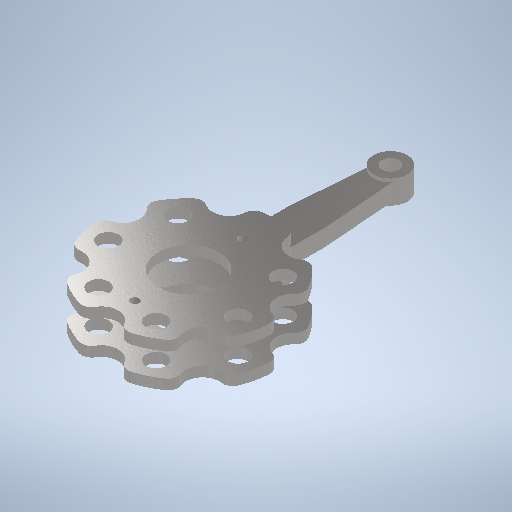
# Autodesk Inventor part: ring
Saved by Autodesk Inventor 2025 (Build 290162010, 162A)
## iProperties
Created: 2024-03-13
Part Number: ring
Material: Stahl, galvanisiert
Document SubType Name: Modeling
Designer: ffogue
Density: 7.85 g/cm^3
Appearance: Galvanisiert
Author: ffogue
Autodesk Inventor part; units mm, degrees
note: some values were not read from the file. Chosen so that the rebuilt part matches the saved one: direction of "Bohrung4"; direction of "Bohrung5"; direction of "Bohrung9"; direction of "Bohrung8".
sketch "Skizze13" plane through (0, 0, 0) normal (0, 1, 0) x (-1, 0, 0)
  line L0 (-5, 6.5) -> (5, 6.5)
  line L1 (5, 6.5) -> (5, -6.5)
  line L2 (5, -6.5) -> (-5, -6.5)
  line L3 (-5, -6.5) -> (-5, 6.5)
  line L4 (-5, 6.5) -> (5, -6.5) construction
  line L5 (5, 6.5) -> (-5, -6.5) construction
  point P0 (0, 0)
  point P1 (0, -6.5)
  dimension "d62" = 13
  dimension "d63" = 10
  constraints: 12 end point, 3 midpoint, 2 parallel, 1 horizontal, 1 perpendicular
  measures "d62" distance from line of point (0, -6.5) L0
  measures "d63" distance between parallel lines of L3 L1
extrude "Extrusion7" add sketch "Skizze13" along normal blind 5
ref_plane "Arbeitsebene3" through (0, 0, 0) normal (0, 0, 1) x (1, 0, 0)
sketch "Skizze14" plane through (0, 0, 0) normal (0, 0, 1) x (1, 0, 0)
  circle A0 centre (0, -20.5147) radius 26
  point P0 (0, 0)
  point P1 (-5, 5)
  point P2 (5, 5)
  dimension "d68" = 52
  constraints: 2 point on circle, 1 centre point
  measures "d68" diameter of A0
extrude "Extrusion8" add sketch "Skizze14" along normal mid plane 13
ref_plane "Arbeitsebene8" through (0, 0, 0) normal (0, 0, 1) x (1, 0, 0)
sketch "Skizze16" plane through (0, 5, 0) normal (0, 0, 1) x (1, 0, 0)
  line L0 (-5.4606, -0.0946) -> (-5.4606, 9.9054)
  line L1 (5.4606, -0.0946) -> (5.4606, 9.9054)
  line L2 (-5.4606, 9.9054) -> (-3.5, 34.4853)
  line L3 (-3.5, 34.4853) -> (3.5, 34.4853)
  line L4 (3.5, 34.4853) -> (5.4606, 9.9054)
  circle A0 centre (0, -25.5147) radius 26 projected
  line L5 (-5.4606, -0.0946) -> (5.4606, -0.0946)
  point P0 (0, 34.4853)
  point P1 (0, 0)
  point P2 (0, -0.0946)
  dimension "d75" = 7
  dimension "d76" = 60
  dimension "d77" = 175.44
  dimension "d153" = 10
  constraints: 13 end point, 2 horizontal, 2 midpoint, 2 vertical, 2 vertical alignment, 1 equal length, 1 horizontal alignment, 2 other
  measures "d75" distance of L2.end L3.end
  measures "d76" distance from line of point (0, -25.515) L3
  measures "d77" angle of L1 L4
  measures "d153" distance of L0.start L0.end
extrude "Extrusion10" add sketch "Skizze16" along normal mid plane 5 contours L0 L2 L3 L4 L1 A0 | A0 L5 picked at (-0.6108, 0.0772)
ref_plane "Arbeitsebene9" through (0, 0, 0) normal (0, 0, 1) x (1, 0, 0)
sketch "Skizze17" plane through (0, -20.5147, 0) normal (0, 0, 1) x (1, 0, 0)
  circle A0 centre (0, 60) radius 5
  line L0 (-3.5, 60) -> (3.5, 60) projected
  point P0 (0, 20.5147)
  dimension "d129" = 10
  constraints: 1 coincident, 1 horizontal alignment, 1 midpoint, 1 other
extrude "Extrusion11" add sketch "Skizze17" along normal mid plane 7
sketch "Skizze18" plane through (0, -20.5147, 6.5) normal (0, 0, 1) x (1, 0, 0)
  circle A0 centre (0, 60) radius 5 projected
  point P0 (0, 20.5147)
  point P1 (0, 60)
  point P2 (3.5, 60)
  point P3 (-3.5, 60)
  point P4 (3.7626, 56.7072)
  point P5 (-3.7626, 56.7072)
  constraints: 1 coincident
hole "Bohrung4" at (0, 39.4853, 6.5) direction (0, 0, -1) diameter 5 depth 13
sketch "Skizze22" plane through (0, -20.5147, 6.5) normal (0, 0, 1) x (1, 0, 0)
  circle A0 centre (0, 0) radius 26 projected
  point P0 (0, 20.5147)
  point P1 (-5, 25.5147)
  point P2 (5, 25.5147)
  constraints: 1 coincident
hole "Bohrung5" at (0, -20.5147, 6.5) direction (0, 0, -1) diameter 18 depth 13
sketch "Skizze19" plane through (0, -20.5147, 6.5) normal (0, 0, 1) x (1, 0, 0)
  circle A0 centre (0, 0) radius 26 projected
  arc A1 (4.9768, -25.5192) -> (-4.9768, -25.5192) centre (0, -26) ccw
  point P0 (0, 20.5147)
  point P1 (0, -21)
  dimension "d90" = 21
  dimension "d91" = 5
  constraints: 5 point on circle, 1 centre point, 1 vertical alignment
  measures "d90" distance of A0.centre point (0, -21)
  measures "d91" radius of A1
extrude "Extrusion12" cut sketch "Skizze19" against normal up to surface (13 mm away) contours A1 A0 picked at (0, -24.2976)
fillet "Rundung3" radius 3 4 edges at (-4.9768, -46.0339, 3.25) (4.9768, -46.0339, 3.25) (4.9768, -46.0339, -3.25) (-4.9768, -46.0339, -3.25)
pattern_circular "Runde Anordnung5" count 7 over 360 about axis through (0, -20.5147, 0) along (0, 0, 1) of "Extrusion12", "Rundung3"
ref_plane "Arbeitsebene5" through (0, -52, 0) normal (0, -1, 0) x (1, 0, 0)
sketch "Skizze27" plane through (0, -46.5147, 6.5) normal (0, 0, 1) x (1, 0, 0)
  arc A0 (-15.6582, 8.0015) -> (-14.5334, 4.4413) centre (-12.8565, 6.9288) ccw projected
  arc A1 (-14.5334, 4.4413) -> (-7.7939, 1.1957) centre (0, 26) ccw projected
  arc A2 (-7.7939, 1.1957) -> (-4.3091, 2.5361) centre (-6.8946, 4.0577) ccw projected
  arc A3 (4.3091, 2.5361) -> (-4.3091, 2.5361) centre (0, 0) ccw projected
  arc A4 (4.3091, 2.5361) -> (7.7939, 1.1957) centre (6.8946, 4.0577) ccw projected
  arc A5 (7.7939, 1.1957) -> (14.5334, 4.4413) centre (0, 26) ccw projected
  arc A6 (14.5334, 4.4413) -> (15.6582, 8.0015) centre (12.8565, 6.9288) ccw projected
  arc A7 (21.0315, 14.7395) -> (15.6582, 8.0015) centre (20.3276, 9.7893) ccw projected
  arc A8 (21.0315, 14.7395) -> (24.2522, 16.6282) centre (21.4539, 17.7096) ccw projected
  arc A9 (24.2522, 16.6282) -> (25.9167, 23.921) centre (0, 26) ccw projected
  arc A10 (25.9167, 23.921) -> (23.8345, 27.0201) centre (22.9264, 24.1609) ccw projected
  arc A11 (21.9168, 35.4223) -> (23.8345, 27.0201) centre (25.3481, 31.7855) ccw projected
  arc A12 (21.9168, 35.4223) -> (22.4482, 39.1179) centre (19.858, 37.6043) ccw projected
  arc A13 (22.4482, 39.1179) -> (17.7842, 44.9663) centre (0, 26) ccw projected
  arc A14 (17.7842, 44.9663) -> (14.063, 45.2706) centre (15.7322, 42.7779) ccw projected
  arc A15 (6.2983, 49.0099) -> (14.063, 45.2706) centre (11.281, 49.4252) ccw projected
  arc A16 (6.2983, 49.0099) -> (3.7402, 51.7296) centre (3.3086, 48.7608) ccw projected
  arc A17 (3.7402, 51.7296) -> (-3.7402, 51.7296) centre (0, 26) ccw projected
  arc A18 (-3.7402, 51.7296) -> (-6.2983, 49.0099) centre (-3.3086, 48.7608) ccw projected
  arc A19 (-14.063, 45.2706) -> (-6.2983, 49.0099) centre (-11.281, 49.4252) ccw projected
  arc A20 (-14.063, 45.2706) -> (-17.7842, 44.9663) centre (-15.7322, 42.7779) ccw projected
  arc A21 (-17.7842, 44.9663) -> (-22.4482, 39.1179) centre (0, 26) ccw projected
  arc A22 (-22.4482, 39.1179) -> (-21.9168, 35.4223) centre (-19.858, 37.6043) ccw projected
  arc A23 (-23.8345, 27.0201) -> (-21.9168, 35.4223) centre (-25.3481, 31.7855) ccw projected
  arc A24 (-23.8345, 27.0201) -> (-25.9167, 23.921) centre (-22.9264, 24.1609) ccw projected
  arc A25 (-25.9167, 23.921) -> (-24.2522, 16.6282) centre (0, 26) ccw projected
  arc A26 (-24.2522, 16.6282) -> (-21.0315, 14.7395) centre (-21.4539, 17.7096) ccw projected
  arc A27 (-15.6582, 8.0015) -> (-21.0315, 14.7395) centre (-20.3276, 9.7893) ccw projected
  circle A28 centre (0, 26) radius 9 projected
  line L0 (0, 26) -> (-20.3276, 42.2107) construction
  circle A29 centre (0, 26) radius 20 construction
  point P0 (0, 46.5147)
  point P1 (-15.6366, 38.4698)
  dimension "d144" = 40
  constraints: 2 end point, 1 coincident, 1 point on circle, 1 point on line, 3 other
hole "Bohrung9" at (-15.6366, -8.0449, 6.5) direction (0, 0, -1) diameter 6 depth 13
pattern_circular "Runde Anordnung6" count 6 over 256 about axis through (0, -20.5147, -99.1125) along (0, 0, 1) of "Bohrung9"
sketch "Skizze25" plane through (0, 39.4853, 6.5) normal (0, 0, 1) x (1, 0, 0)
  line L0 (-30.4283, -60) -> (44.8927, -60) construction
  circle A0 centre (0, -60) radius 9 projected
  point P0 (0, -39.4853)
  point P1 (0, -44)
  point P2 (0, -76)
  dimension "d137" = 32
  constraints: 2 end point, 2 vertical alignment, 1 horizontal, 1 point on line, 1 symmetric about line
  measures "d137" distance of point (0, -76) point (0, -44)
hole "Bohrung8" at (0, -4.5147, 6.5) at (0, -36.5147, 6.5) direction (0, 0, -1) diameter 2.459 depth 13 thread size "M3x0.5" class "6H" standard "ISO Metric profile"
sketch "Skizze20" plane through (0, -52, 0) normal (0, -1, 0) x (1, 0, 0)
  line L0 (-26, 3.5) -> (26, 3.5)
  line L1 (26, 3.5) -> (26, -3.5)
  line L2 (26, -3.5) -> (-26, -3.5)
  line L3 (-26, -3.5) -> (-26, 3.5)
  line L4 (0, 0) -> (0, 4.767) construction
  point P0 (-26, 0)
  point P1 (26, 0)
  dimension "d100" = 7
  dimension "d101" = 52
  constraints: 10 end point, 2 midpoint, 2 parallel, 1 horizontal, 1 horizontal alignment, 1 perpendicular, 1 vertical, 1 other
  measures "d100" distance between parallel lines of L2 L0
  measures "d101" distance between parallel lines of L1 L3
extrude "Extrusion13" cut sketch "Skizze20" against normal blind 52
